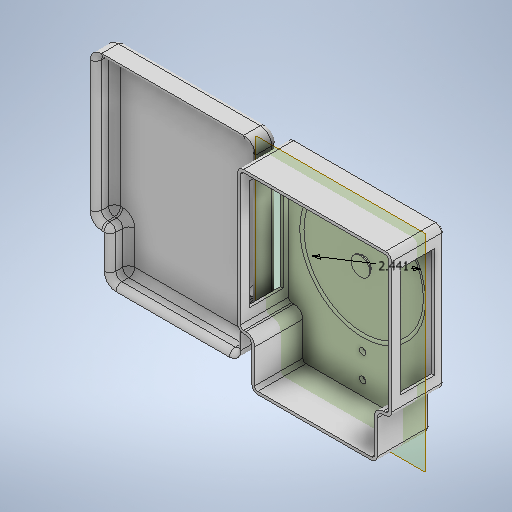
# Autodesk Inventor part: WireRewindShellyBoi
Saved by Autodesk Inventor 2025.1 (Build 291241000, 241)
## iProperties
Created: 2024-10-25
Part Number: WireRewindShellyBoi
Material: Generic
Document SubType Name: Modeling
Designer: ishaa
Density: 1 g/cm^3
Appearance: Default
Author: ishaa
Autodesk Inventor part; units mm, degrees
ref_plane "YZ Plane" through (0, 0, 0) normal (1, 0, 0) x (0, 1, 0)
ref_plane "XZ Plane" through (0, 0, 0) normal (0, 1, 0) x (-1, 0, 0)
ref_plane "XY Plane" through (0, 0, 0) normal (0, 0, 1) x (1, 0, 0)
sketch "Sketch1" plane through (0, 0, 0) normal (0, 0, 1) x (1, 0, 0)
  circle A0 centre (0, 0) radius 31 construction
  dimension "d0" = 62
  constraints: 1 centre point, 1 coincident
  measures "d0" diameter of A0
sketch "Sketch2" plane through (0, 0, 0) normal (0, 0, 1) x (1, 0, 0)
  line L0 (-40.6616, 34.3864) -> (-40.6616, 0)
  line L1 (-144.6853, 0) -> (57.3144, 0) construction
  line L2 (0, 84.9629) -> (0, -74.7936) construction
  line L3 (-40.6616, -34.3864) -> (-40.6616, 0)
  line L4 (40.6616, 34.3864) -> (40.6616, 0)
  line L5 (40.6616, -34.3864) -> (40.6616, 0)
  line L6 (-37.4866, -37.5614) -> (-36.3155, -37.5614)
  line L7 (-33.1405, -40.7364) -> (-33.1405, -58.5164)
  line L8 (-29.9655, -61.6914) -> (0, -61.6914)
  line L9 (-37.4866, 37.5614) -> (0, 37.5614)
  line L10 (37.4866, -37.5614) -> (36.3155, -37.5614)
  line L11 (33.1405, -40.7364) -> (33.1405, -58.5164)
  line L12 (29.9655, -61.6914) -> (0, -61.6914)
  line L13 (37.4866, 37.5614) -> (0, 37.5614)
  arc A0 (36.3155, -37.5614) -> (33.1405, -40.7364) centre (36.3155, -40.7364) ccw
  arc A1 (-33.1405, -40.7364) -> (-36.3155, -37.5614) centre (-36.3155, -40.7364) ccw
  arc A2 (-33.1405, -58.5164) -> (-29.9655, -61.6914) centre (-29.9655, -58.5164) ccw
  arc A3 (29.9655, -61.6914) -> (33.1405, -58.5164) centre (29.9655, -58.5164) ccw
  arc A4 (40.6616, 34.3864) -> (37.4866, 37.5614) centre (37.4866, 34.3864) ccw
  arc A5 (-37.4866, 37.5614) -> (-40.6616, 34.3864) centre (-37.4866, 34.3864) ccw
  arc A6 (37.4866, -37.5614) -> (40.6616, -34.3864) centre (37.4866, -34.3864) ccw
  arc A7 (-40.6616, -34.3864) -> (-37.4866, -37.5614) centre (-37.4866, -34.3864) ccw
  point P0 (0, 0)
  point P1 (-40.6616, 37.5614)
  point P2 (-40.6616, -37.5614)
  point P3 (40.6616, 37.5614)
  point P4 (40.6616, -37.5614)
  point P5 (-33.1405, -37.5614)
  point P6 (-33.1405, -61.6914)
  point P7 (33.1405, -37.5614)
  point P8 (33.1405, -61.6914)
  dimension "d1" = 24.13
  dimension "d2" = 3.175
  dimension "d3" = 3.175
  dimension "d4" = 3.175
  constraints: 28 end point, 18 point on line, 16 point on circle, 16 tangent, 8 centre point, 6 symmetric about line, 5 equal radius, 3 horizontal, 2 perpendicular, 2 vertical
  measures "d1" distance of point (-33.14, -37.561) point (-33.14, -61.691)
  measures "d2" radius of A0
  measures "d3" radius of A1
  measures "d4" radius of A2
extrude "Extrusion1" add sketch "Sketch2" along normal blind 2
sketch "Sketch3" plane through (0, 0, 2) normal (0, 0, 1) x (1, 0, 0)
  line L0 (-40.6616, 34.3864) -> (-40.6616, -34.3864) projected
  arc A0 (-40.6616, -34.3864) -> (-37.4866, -37.5614) centre (-37.4866, -34.3864) ccw projected
  line L1 (-37.4866, -37.5614) -> (-36.3155, -37.5614) projected
  arc A1 (-33.1405, -40.7364) -> (-36.3155, -37.5614) centre (-36.3155, -40.7364) ccw projected
  line L2 (-33.1405, -40.7364) -> (-33.1405, -58.5164) projected
  arc A2 (-33.1405, -58.5164) -> (-29.9655, -61.6914) centre (-29.9655, -58.5164) ccw projected
  line L3 (-29.9655, -61.6914) -> (29.9655, -61.6914) projected
  arc A3 (29.9655, -61.6914) -> (33.1405, -58.5164) centre (29.9655, -58.5164) ccw projected
  line L4 (33.1405, -58.5164) -> (33.1405, -40.7364) projected
  arc A4 (36.3155, -37.5614) -> (33.1405, -40.7364) centre (36.3155, -40.7364) ccw projected
  line L5 (36.3155, -37.5614) -> (37.4866, -37.5614) projected
  arc A5 (37.4866, -37.5614) -> (40.6616, -34.3864) centre (37.4866, -34.3864) ccw projected
  line L6 (40.6616, -34.3864) -> (40.6616, 34.3864) projected
  arc A6 (40.6616, 34.3864) -> (37.4866, 37.5614) centre (37.4866, 34.3864) ccw projected
  line L7 (37.4866, 37.5614) -> (-37.4866, 37.5614) projected
  arc A7 (-37.4866, 37.5614) -> (-40.6616, 34.3864) centre (-37.4866, 34.3864) ccw projected
  line L8 (-37.4866, 36.0614) -> (37.4866, 36.0614)
  arc A8 (39.1616, 34.3864) -> (37.4866, 36.0614) centre (37.4866, 34.3864) ccw
  line L9 (39.1616, 34.3864) -> (39.1616, -34.3864)
  arc A9 (37.4866, -36.0614) -> (39.1616, -34.3864) centre (37.4866, -34.3864) ccw
  line L10 (37.4866, -36.0614) -> (36.3155, -36.0614)
  arc A10 (36.3155, -36.0614) -> (31.6405, -40.7364) centre (36.3155, -40.7364) ccw
  line L11 (31.6405, -40.7364) -> (31.6405, -58.5164)
  arc A11 (29.9655, -60.1914) -> (31.6405, -58.5164) centre (29.9655, -58.5164) ccw
  line L12 (29.9655, -60.1914) -> (-29.9655, -60.1914)
  arc A12 (-31.6405, -58.5164) -> (-29.9655, -60.1914) centre (-29.9655, -58.5164) ccw
  line L13 (-31.6405, -58.5164) -> (-31.6405, -40.7364)
  arc A13 (-31.6405, -40.7364) -> (-36.3155, -36.0614) centre (-36.3155, -40.7364) ccw
  line L14 (-36.3155, -36.0614) -> (-37.4866, -36.0614)
  arc A14 (-39.1616, -34.3864) -> (-37.4866, -36.0614) centre (-37.4866, -34.3864) ccw
  line L15 (-39.1616, -34.3864) -> (-39.1616, 34.3864)
  arc A15 (-37.4866, 36.0614) -> (-39.1616, 34.3864) centre (-37.4866, 34.3864) ccw
  point P0 (0, 0)
  dimension "d7" = 1.5
  constraints: 16 end point, 16 point on circle, 8 centre point, 15 other
  measures "d7" distance between parallel lines of L7 L8
extrude "Extrusion2" add sketch "Sketch3" along normal blind 25.4
sketch "Sketch4" plane through (-29.9655, -61.6914, 0) normal (0, -1, 0) x (1, 0, 0)
  line L0 (0, 0) -> (0, 27.4) construction
  line L1 (0, 13.7) -> (59.931, 13.7) construction
  line L2 (59.931, 0) -> (59.931, 27.4) construction
  point P0 (29.9655, 0)
  constraints: 2 end point, 2 midpoint
ref_plane "Work Plane1" through (-29.9655, -61.6914, 13.7) normal (0, 0, -1) x (1, 0, 0)
sketch "Sketch5" plane through (-40.6616, -34.3864, 0) normal (-1, 0, 0) x (0, 0, 1)
  line L0 (22.4984, 63.4868) -> (4.8171, 63.4868)
  line L1 (4.8171, 63.4868) -> (4.8171, 5.5154)
  line L2 (4.8171, 5.5154) -> (22.4984, 5.5154)
  line L3 (22.4984, 5.5154) -> (22.4984, 63.4868)
  line L4 (0, 68.7728) -> (0, 0) projected
  point P0 (0, 34.3864)
  dimension "d11" = 4.8171
  dimension "d12" = 57.9714
  dimension "d13" = 17.6813
  dimension "d14" = 5.286
  constraints: 8 end point, 2 parallel, 1 horizontal, 1 perpendicular
  measures "d11" distance between parallel lines of L4 L1
  measures "d12" distance between parallel lines of L2 L0
  measures "d13" distance from line of L0.end L3
  measures "d14" distance from line of L4.start L0
extrude "Extrusion3" cut sketch "Sketch5" against normal blind 844073.3515
sketch "Sketch6" plane through (0, 0, 2) normal (0, 0, 1) x (1, 0, 0)
  line L0 (-29.9655, -60.1914) -> (29.9655, -60.1914) construction
  line L1 (0, -60.1914) -> (0, 34.6609) construction
  circle A0 centre (0, -52.6439) radius 1.7
  circle A1 centre (0, -39.4763) radius 1.7
  point P0 (0, 0)
  dimension "d17" = 3.4
  dimension "d26" = 3.4
  dimension "d29" = 94.8524
  dimension "d30" = 20.7151
  dimension "d31" = 7.5475
  dimension "d32" = 0
  constraints: 2 centre point, 2 end point, 1 midpoint, 1 point on line, 1 vertical
  measures "d17" diameter of A0
  measures "d26" diameter of A1
  measures "d29" distance from line of L1.end L0
  measures "d30" distance from line of A1.centre L0
  measures "d31" distance from line of A0.centre L0
  measures "d32" distance from line of A1.centre L1
extrude "Extrusion4" cut sketch "Sketch6" against normal blind 844073.3515
sketch "Sketch7" plane through (0, 0, 2) normal (0, 0, 1) x (1, 0, 0)
  circle A0 centre (0, 0) radius 31.5
  dimension "d22" = 63
  constraints: 1 centre point, 1 coincident
  measures "d22" diameter of A0
extrude "Extrusion5" cut sketch "Sketch7" against normal blind 0.5
fillet "Fillet1" radius 3.175 1 edges at (-31.5, 0, 2)
sketch "Sketch8" plane through (0, 0, 1.5) normal (0, 0, 1) x (1, 0, 0)
  point P0 (0, 0)
sketch "Sketch9" plane through (0, 0, 1.5) normal (0, 0, 1) x (1, 0, 0)
  circle A0 centre (0, 0) radius 4
  dimension "d33" = 8
  constraints: 1 centre point, 1 coincident
  measures "d33" diameter of A0
extrude "Extrusion6" add sketch "Sketch9" along normal blind 1.5
sketch "Sketch10" plane through (0, 0, 3) normal (0, 0, 1) x (1, 0, 0)
  circle A0 centre (0, 0) radius 4 projected
  circle A1 centre (0, 0) radius 4.9243
  constraints: 1 centre point
extrude "Extrusion7" add sketch "Sketch10" along normal mid plane 0.5 contours A0 | A1
sketch "Sketch11" plane through (-90.3868, -2.7855, 0) normal (0, 0, 1) x (1, 0, 0)
  line L0 (-40.6616, 34.3864) -> (-40.6616, 0)
  line L1 (-144.6853, 0) -> (57.3144, 0) construction
  line L2 (0, 84.9629) -> (0, -74.7936) construction
  line L3 (-40.6616, -34.3864) -> (-40.6616, 0)
  line L4 (40.6616, 34.3864) -> (40.6616, 0)
  line L5 (40.6616, -34.3864) -> (40.6616, 0)
  line L6 (-37.4866, -37.5614) -> (-36.3155, -37.5614)
  line L7 (-33.1405, -40.7364) -> (-33.1405, -58.5164)
  line L8 (-29.9655, -61.6914) -> (0, -61.6914)
  line L9 (-37.4866, 37.5614) -> (0, 37.5614)
  line L10 (37.4866, 37.5614) -> (0, 37.5614)
  line L11 (37.4866, -37.5614) -> (36.3155, -37.5614)
  line L12 (33.1405, -40.7364) -> (33.1405, -58.5164)
  line L13 (29.9655, -61.6914) -> (0, -61.6914)
  arc A0 (36.3155, -37.5614) -> (33.1405, -40.7364) centre (36.3155, -40.7364) ccw
  arc A1 (-33.1405, -40.7364) -> (-36.3155, -37.5614) centre (-36.3155, -40.7364) ccw
  arc A2 (-33.1405, -58.5164) -> (-29.9655, -61.6914) centre (-29.9655, -58.5164) ccw
  arc A3 (29.9655, -61.6914) -> (33.1405, -58.5164) centre (29.9655, -58.5164) ccw
  arc A4 (40.6616, 34.3864) -> (37.4866, 37.5614) centre (37.4866, 34.3864) ccw
  arc A5 (-37.4866, 37.5614) -> (-40.6616, 34.3864) centre (-37.4866, 34.3864) ccw
  arc A6 (37.4866, -37.5614) -> (40.6616, -34.3864) centre (37.4866, -34.3864) ccw
  arc A7 (-40.6616, -34.3864) -> (-37.4866, -37.5614) centre (-37.4866, -34.3864) ccw
  point P0 (0, 0)
  point P1 (-40.6616, 37.5614)
  point P2 (-40.6616, -37.5614)
  point P3 (40.6616, 37.5614)
  point P4 (40.6616, -37.5614)
  point P5 (-33.1405, -37.5614)
  point P6 (-33.1405, -61.6914)
  point P7 (33.1405, -37.5614)
  point P8 (33.1405, -61.6914)
  dimension "d41" = 24.13
  dimension "d40" = 3.175
  dimension "d39" = 3.175
  dimension "d38" = 3.175
  constraints: 28 end point, 18 point on line, 16 point on circle, 16 tangent, 8 centre point, 6 symmetric about line, 5 equal radius, 3 horizontal, 2 perpendicular, 2 vertical
  measures "d41" distance of point (-33.14, -37.561) point (-33.14, -61.691)
  measures "d40" radius of A0
  measures "d39" radius of A1
  measures "d38" radius of A2
extrude "Extrusion8" add sketch "Sketch11" along normal blind 2 separate body
sketch "Sketch12" plane through (-90.3868, -2.7855, 2) normal (0, 0, 1) x (1, 0, 0)
  line L0 (-40.6616, 34.3864) -> (-40.6616, -34.3864) projected
  arc A0 (-40.6616, -34.3864) -> (-37.4866, -37.5614) centre (-37.4866, -34.3864) ccw projected
  line L1 (-37.4866, -37.5614) -> (-36.3155, -37.5614) projected
  arc A1 (-33.1405, -40.7364) -> (-36.3155, -37.5614) centre (-36.3155, -40.7364) ccw projected
  line L2 (-33.1405, -40.7364) -> (-33.1405, -58.5164) projected
  arc A2 (-33.1405, -58.5164) -> (-29.9655, -61.6914) centre (-29.9655, -58.5164) ccw projected
  line L3 (-29.9655, -61.6914) -> (29.9655, -61.6914) projected
  arc A3 (29.9655, -61.6914) -> (33.1405, -58.5164) centre (29.9655, -58.5164) ccw projected
  line L4 (33.1405, -58.5164) -> (33.1405, -40.7364) projected
  arc A4 (36.3155, -37.5614) -> (33.1405, -40.7364) centre (36.3155, -40.7364) ccw projected
  line L5 (36.3155, -37.5614) -> (37.4866, -37.5614) projected
  arc A5 (37.4866, -37.5614) -> (40.6616, -34.3864) centre (37.4866, -34.3864) ccw projected
  line L6 (40.6616, -34.3864) -> (40.6616, 34.3864) projected
  arc A6 (40.6616, 34.3864) -> (37.4866, 37.5614) centre (37.4866, 34.3864) ccw projected
  line L7 (37.4866, 37.5614) -> (-37.4866, 37.5614) projected
  arc A7 (-37.4866, 37.5614) -> (-40.6616, 34.3864) centre (-37.4866, 34.3864) ccw projected
  line L8 (-37.4866, 40.5084) -> (37.4866, 40.5084)
  arc A8 (43.6086, 34.3864) -> (37.4866, 40.5084) centre (37.4866, 34.3864) ccw
  line L9 (43.6086, 34.3864) -> (43.6086, -34.3864)
  arc A9 (37.4866, -40.5084) -> (43.6086, -34.3864) centre (37.4866, -34.3864) ccw
  line L10 (37.4866, -40.5084) -> (36.3155, -40.5084)
  arc A10 (36.3155, -40.5084) -> (36.0875, -40.7364) centre (36.3155, -40.7364) ccw
  line L11 (36.0875, -40.7364) -> (36.0875, -58.5164)
  arc A11 (29.9655, -64.6384) -> (36.0875, -58.5164) centre (29.9655, -58.5164) ccw
  line L12 (29.9655, -64.6384) -> (-29.9655, -64.6384)
  arc A12 (-36.0875, -58.5164) -> (-29.9655, -64.6384) centre (-29.9655, -58.5164) ccw
  line L13 (-36.0875, -58.5164) -> (-36.0875, -40.7364)
  arc A13 (-36.0875, -40.7364) -> (-36.3155, -40.5084) centre (-36.3155, -40.7364) ccw
  line L14 (-36.3155, -40.5084) -> (-37.4866, -40.5084)
  arc A14 (-43.6086, -34.3864) -> (-37.4866, -40.5084) centre (-37.4866, -34.3864) ccw
  line L15 (-43.6086, -34.3864) -> (-43.6086, 34.3864)
  arc A15 (-37.4866, 40.5084) -> (-43.6086, 34.3864) centre (-37.4866, 34.3864) ccw
  point P0 (90.3868, 2.7855)
  constraints: 16 end point, 16 point on circle, 8 centre point, 15 other
extrude "Extrusion9" add sketch "Sketch12" along normal blind 10 and the other way blind 2
fillet "Fillet2" radius 3.175 32 edges at (-58.1763, -63.547, 12) (-90.3868, -64.4769, 12) (-122.5974, -63.547, 12) (-123.5273, -52.4119, 12) (-124.4572, -41.2768, 12) (-127.2879, -40.3469, 12) (-130.1185, -39.417, 12) (-131.0484, -2.7855, 12) (-130.1185, 33.846, 12) (-90.3868, 34.7759, 12) (-50.6552, 33.846, 12) (-49.7253, -2.7855, 12) (-50.6552, -39.417, 12) (-53.4858, -40.3469, 12) (-56.3164, -41.2768, 12) (-57.2463, -52.4119, 12) (-53.4858, -40.3469, 2) (-50.6552, -39.417, 2) (-49.7253, -2.7855, 2) (-50.6552, 33.846, 2) (-90.3868, 34.7759, 2) (-130.1185, 33.846, 2) (-131.0484, -2.7855, 2) (-130.1185, -39.417, 2) (-127.2879, -40.3469, 2) (-124.4572, -41.2768, 2) (-123.5273, -52.4119, 2) (-122.5974, -63.547, 2) (-90.3868, -64.4769, 2) (-58.1763, -63.547, 2) (-57.2463, -52.4119, 2) (-56.3164, -41.2768, 2)
fillet "Fillet3" radius 3.175 16 edges at (-124.6812, -65.6308, 0) (-126.4743, -52.4119, 0) (-126.5411, -43.3607, 0) (-127.2879, -43.2939, 0) (-132.2023, -41.5008, 0) (-133.9954, -2.7855, 0) (-132.2023, 35.9298, 0) (-90.3868, 37.7229, 0) (-48.5713, 35.9298, 0) (-46.7783, -2.7855, 0) (-48.5713, -41.5008, 0) (-53.4858, -43.2939, 0) (-54.2326, -43.3607, 0) (-54.2993, -52.4119, 0) (-56.0924, -65.6308, 0) (-90.3868, -67.4239, 0)
fillet "Fillet4" radius 1 16 edges at (32.2105, -60.7615, 0) (33.1405, -49.6264, 0) (34.0704, -38.4913, 0) (36.901, -37.5614, 0) (39.7316, -36.6315, 0) (40.6616, 0, 0) (39.7316, 36.6315, 0) (0, 37.5614, 0) (-39.7316, 36.6315, 0) (-40.6616, 0, 0) (-39.7316, -36.6315, 0) (-36.901, -37.5614, 0) (-34.0704, -38.4913, 0) (-33.1405, -49.6264, 0) (-32.2105, -60.7615, 0) (0, -61.6914, 0)
body "Solid1"
